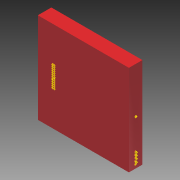
# Autodesk Inventor part: xM
Saved by Autodesk Inventor 2011 SP1 (Build 150282100, 282)
## iProperties
Created: 2011-06-13
Part Number: xM
Document SubType Name: Modeling
Designer: Andrew G. Meyer
Mass: 92.5046 g
Surface Area: 189.909 cm^2
Volume: 92.5046 cm^3
Density: 1 g/cm^3
Author: Andrew G. Meyer
Autodesk Inventor part; units mm, degrees
ref_plane "YZ Plane" through (0, 0, 0) normal (1, 0, 0) x (0, 1, 0)
ref_plane "XZ Plane" through (0, 0, 0) normal (0, 1, 0) x (-1, 0, 0)
ref_plane "XY Plane" through (0, 0, 0) normal (0, 0, 1) x (1, 0, 0)
sketch "Sketch1" plane through (0, 0, 0) normal (0, 0, 1) x (1, 0, 0)
  line L0 (-22.1557, 68.2637) -> (63.4423, 68.2637)
  line L1 (63.4423, 68.2637) -> (63.4423, -16.8263)
  line L2 (63.4423, -16.8263) -> (-22.1557, -16.8263)
  line L3 (-22.1557, -16.8263) -> (-22.1557, 68.2637)
  point P0 (0, 0)
  dimension "d0" = 85.09
  dimension "d1" = 85.598
  constraints: 8 end point, 2 parallel, 1 horizontal, 1 perpendicular
  measures "d0" distance of L2.end L0.start
  measures "d1" distance of L1.end L2.end
extrude "Extrusion1" add sketch "Sketch1" along normal blind 12.7
sketch "Sketch2" plane through (0, 0, 12.7) normal (0, 0, 1) x (1, 0, 0)
  line L0 (-22.1557, 68.2637) -> (63.4423, 68.2637) projected
  line L1 (-22.1557, -16.8263) -> (-22.1557, 68.2637) projected
  line L2 (63.4423, -16.8263) -> (-22.1557, -16.8263) projected
  line L3 (-9.4557, 36.5137) -> (-6.2807, 36.5137)
  line L4 (-6.2807, 36.5137) -> (-6.2807, 14.9237)
  line L5 (-6.2807, 14.9237) -> (-9.4557, 14.9237)
  line L6 (-9.4557, 14.9237) -> (-9.4557, 36.5137)
  point P0 (0, 0)
  dimension "d4" = 31.75
  dimension "d5" = 31.75
  dimension "d6" = 12.7
  dimension "d7" = 3.175
  constraints: 8 end point, 2 parallel, 1 horizontal, 1 perpendicular
  measures "d4" distance between parallel lines of L0 L3
  measures "d5" distance between parallel lines of L2 L5
  measures "d6" distance between parallel lines of L1 L6
  measures "d7" distance of L4.end L5.end
extrude "Extrusion2" cut sketch "Sketch2" against normal blind 0.254
sketch "Sketch3" plane through (0, 0, 12.446) normal (0, 0, 1) x (1, 0, 0)
  line L0 (-9.4557, 36.5137) -> (-9.4557, 14.9237) projected
  line L1 (-9.4557, 14.9237) -> (-6.2807, 14.9237) projected
  line L2 (-6.2807, 14.9237) -> (-7.7412, 14.9237)
  line L3 (-7.7412, 14.9237) -> (-7.7412, 16.3842)
  line L4 (-7.7412, 16.3842) -> (-6.2807, 16.3842)
  line L5 (-6.2807, 16.3842) -> (-6.2807, 14.9237)
  line L6 (-9.4557, 16.3842) -> (-7.9952, 16.3842)
  line L7 (-7.9952, 16.3842) -> (-7.9952, 14.9237)
  line L8 (-7.9952, 14.9237) -> (-9.4557, 14.9237)
  line L9 (-9.4557, 14.9237) -> (-9.4557, 16.3842)
  line L10 (-6.2807, 16.5112) -> (-7.7412, 16.5112)
  line L11 (-7.7412, 16.5112) -> (-7.7412, 17.9717)
  line L12 (-7.7412, 17.9717) -> (-6.2807, 17.9717)
  line L13 (-6.2807, 17.9717) -> (-6.2807, 16.5112)
  line L14 (-9.4557, 17.9717) -> (-7.9952, 17.9717)
  line L15 (-7.9952, 17.9717) -> (-7.9952, 16.5112)
  line L16 (-7.9952, 16.5112) -> (-9.4557, 16.5112)
  line L17 (-9.4557, 16.5112) -> (-9.4557, 17.9717)
  line L18 (-6.2807, 18.0987) -> (-7.7412, 18.0987)
  line L19 (-7.7412, 18.0987) -> (-7.7412, 19.5592)
  line L20 (-7.7412, 19.5592) -> (-6.2807, 19.5592)
  line L21 (-6.2807, 19.5592) -> (-6.2807, 18.0987)
  line L22 (-9.4557, 19.5592) -> (-7.9952, 19.5592)
  line L23 (-7.9952, 19.5592) -> (-7.9952, 18.0987)
  line L24 (-7.9952, 18.0987) -> (-9.4557, 18.0987)
  line L25 (-9.4557, 18.0987) -> (-9.4557, 19.5592)
  line L26 (-6.2807, 19.6862) -> (-7.7412, 19.6862)
  line L27 (-7.7412, 19.6862) -> (-7.7412, 21.1467)
  line L28 (-7.7412, 21.1467) -> (-6.2807, 21.1467)
  line L29 (-6.2807, 21.1467) -> (-6.2807, 19.6862)
  line L30 (-9.4557, 21.1467) -> (-7.9952, 21.1467)
  line L31 (-7.9952, 21.1467) -> (-7.9952, 19.6862)
  line L32 (-7.9952, 19.6862) -> (-9.4557, 19.6862)
  line L33 (-9.4557, 19.6862) -> (-9.4557, 21.1467)
  line L34 (-6.2807, 21.2737) -> (-7.7412, 21.2737)
  line L35 (-7.7412, 21.2737) -> (-7.7412, 22.7342)
  line L36 (-7.7412, 22.7342) -> (-6.2807, 22.7342)
  line L37 (-6.2807, 22.7342) -> (-6.2807, 21.2737)
  line L38 (-9.4557, 22.7342) -> (-7.9952, 22.7342)
  line L39 (-7.9952, 22.7342) -> (-7.9952, 21.2737)
  line L40 (-7.9952, 21.2737) -> (-9.4557, 21.2737)
  line L41 (-9.4557, 21.2737) -> (-9.4557, 22.7342)
  line L42 (-6.2807, 22.8612) -> (-7.7412, 22.8612)
  line L43 (-7.7412, 22.8612) -> (-7.7412, 24.3217)
  line L44 (-7.7412, 24.3217) -> (-6.2807, 24.3217)
  line L45 (-6.2807, 24.3217) -> (-6.2807, 22.8612)
  line L46 (-9.4557, 24.3217) -> (-7.9952, 24.3217)
  line L47 (-7.9952, 24.3217) -> (-7.9952, 22.8612)
  line L48 (-7.9952, 22.8612) -> (-9.4557, 22.8612)
  line L49 (-9.4557, 22.8612) -> (-9.4557, 24.3217)
  line L50 (-6.2807, 24.4487) -> (-7.7412, 24.4487)
  line L51 (-7.7412, 24.4487) -> (-7.7412, 25.9092)
  line L52 (-7.7412, 25.9092) -> (-6.2807, 25.9092)
  line L53 (-6.2807, 25.9092) -> (-6.2807, 24.4487)
  line L54 (-9.4557, 25.9092) -> (-7.9952, 25.9092)
  line L55 (-7.9952, 25.9092) -> (-7.9952, 24.4487)
  line L56 (-7.9952, 24.4487) -> (-9.4557, 24.4487)
  line L57 (-9.4557, 24.4487) -> (-9.4557, 25.9092)
  line L58 (-6.2807, 26.0362) -> (-7.7412, 26.0362)
  line L59 (-7.7412, 26.0362) -> (-7.7412, 27.4967)
  line L60 (-7.7412, 27.4967) -> (-6.2807, 27.4967)
  line L61 (-6.2807, 27.4967) -> (-6.2807, 26.0362)
  line L62 (-9.4557, 27.4967) -> (-7.9952, 27.4967)
  line L63 (-7.9952, 27.4967) -> (-7.9952, 26.0362)
  line L64 (-7.9952, 26.0362) -> (-9.4557, 26.0362)
  line L65 (-9.4557, 26.0362) -> (-9.4557, 27.4967)
  line L66 (-6.2807, 27.6237) -> (-7.7412, 27.6237)
  line L67 (-7.7412, 27.6237) -> (-7.7412, 29.0842)
  line L68 (-7.7412, 29.0842) -> (-6.2807, 29.0842)
  line L69 (-6.2807, 29.0842) -> (-6.2807, 27.6237)
  line L70 (-9.4557, 29.0842) -> (-7.9952, 29.0842)
  line L71 (-7.9952, 29.0842) -> (-7.9952, 27.6237)
  line L72 (-7.9952, 27.6237) -> (-9.4557, 27.6237)
  line L73 (-9.4557, 27.6237) -> (-9.4557, 29.0842)
  line L74 (-6.2807, 29.2112) -> (-7.7412, 29.2112)
  line L75 (-7.7412, 29.2112) -> (-7.7412, 30.6717)
  line L76 (-7.7412, 30.6717) -> (-6.2807, 30.6717)
  line L77 (-6.2807, 30.6717) -> (-6.2807, 29.2112)
  line L78 (-9.4557, 30.6717) -> (-7.9952, 30.6717)
  line L79 (-7.9952, 30.6717) -> (-7.9952, 29.2112)
  line L80 (-7.9952, 29.2112) -> (-9.4557, 29.2112)
  line L81 (-9.4557, 29.2112) -> (-9.4557, 30.6717)
  line L82 (-6.2807, 30.7987) -> (-7.7412, 30.7987)
  line L83 (-7.7412, 30.7987) -> (-7.7412, 32.2592)
  line L84 (-7.7412, 32.2592) -> (-6.2807, 32.2592)
  line L85 (-6.2807, 32.2592) -> (-6.2807, 30.7987)
  line L86 (-9.4557, 32.2592) -> (-7.9952, 32.2592)
  line L87 (-7.9952, 32.2592) -> (-7.9952, 30.7987)
  line L88 (-7.9952, 30.7987) -> (-9.4557, 30.7987)
  line L89 (-9.4557, 30.7987) -> (-9.4557, 32.2592)
  line L90 (-6.2807, 32.3862) -> (-7.7412, 32.3862)
  line L91 (-7.7412, 32.3862) -> (-7.7412, 33.8467)
  line L92 (-7.7412, 33.8467) -> (-6.2807, 33.8467)
  line L93 (-6.2807, 33.8467) -> (-6.2807, 32.3862)
  line L94 (-9.4557, 33.8467) -> (-7.9952, 33.8467)
  line L95 (-7.9952, 33.8467) -> (-7.9952, 32.3862)
  line L96 (-7.9952, 32.3862) -> (-9.4557, 32.3862)
  line L97 (-9.4557, 32.3862) -> (-9.4557, 33.8467)
  line L98 (-6.2807, 33.9737) -> (-7.7412, 33.9737)
  line L99 (-7.7412, 33.9737) -> (-7.7412, 35.4342)
  line L100 (-7.7412, 35.4342) -> (-6.2807, 35.4342)
  line L101 (-6.2807, 35.4342) -> (-6.2807, 33.9737)
  line L102 (-9.4557, 35.4342) -> (-7.9952, 35.4342)
  line L103 (-7.9952, 35.4342) -> (-7.9952, 33.9737)
  line L104 (-7.9952, 33.9737) -> (-9.4557, 33.9737)
  line L105 (-9.4557, 33.9737) -> (-9.4557, 35.4342)
  point P0 (0, 0)
  dimension "d10" = 0.254
  dimension "d13" = 1.5875
  constraints: 208 end point, 4 parallel, 3 equal length, 2 horizontal, 2 perpendicular, 2 point on line, 1 vertical, 192 other
  measures "d10" distance between parallel lines of L3 L7
  measures "d13" distance of L6.start L14.start
extrude "Extrusion3" add sketch "Sketch3" along normal blind 0.508
sketch "Sketch4" plane through (63.4423, -16.8263, 0) normal (1, 0, 0) x (0, 0, -1)
  line L0 (-12.7, 85.09) -> (-12.7, 0) projected
  line L1 (0, 0) -> (-12.7, 0) projected
  line L2 (0, 85.09) -> (0, 0) projected
  line L3 (0, 85.09) -> (-12.7, 85.09) projected
  circle A0 centre (-6.35, 42.545) radius 1.05
  circle A1 centre (-6.35, 42.545) radius 0.35
  line L4 (-6.35, 42.545) -> (-6.35, 0) construction
  line L5 (-6.35, 42.545) -> (-6.35, 85.09) construction
  line L6 (-6.35, 42.545) -> (0, 42.545) construction
  line L7 (-6.35, 42.545) -> (-12.7, 42.545) construction
  circle A2 centre (-6.35, 41.845) radius 0.25
  line L8 (-6.35, 41.845) -> (-6.35, 42.195) construction
  line L9 (-6.35, 41.845) -> (-6.35, 41.495) construction
  line L10 (-7.9375, 3.556) -> (-7.9375, 13.8995)
  line L11 (-6.579, 14.856) -> (-5.436, 14.4468)
  line L12 (-4.7625, 13.4902) -> (-4.7625, 3.9652)
  line L13 (-5.436, 3.0087) -> (-6.579, 2.5995)
  arc A3 (-7.9375, 3.556) -> (-6.579, 2.5995) centre (-6.9215, 3.556) ccw
  arc A4 (-5.436, 3.0087) -> (-4.7625, 3.9652) centre (-5.7785, 3.9652) ccw
  arc A5 (-6.579, 14.856) -> (-7.9375, 13.8995) centre (-6.9215, 13.8995) ccw
  arc A6 (-4.7625, 13.4902) -> (-5.436, 14.4468) centre (-5.7785, 13.4902) ccw
  circle A7 centre (-6.9215, 3.556) radius 0.6579
  circle A8 centre (-6.9215, 6.1419) radius 0.6579
  circle A9 centre (-6.9215, 8.7277) radius 0.6579
  circle A10 centre (-6.9215, 13.8995) radius 0.6579
  line L14 (-6.9215, 3.556) -> (-6.9215, 6.1419) construction
  line L15 (-6.9215, 6.1419) -> (-6.9215, 8.7277) construction
  circle A11 centre (-5.7785, 4.8489) radius 0.6579
  circle A12 centre (-6.9215, 11.3136) radius 0.6579
  circle A13 centre (-5.7785, 7.4348) radius 0.6579
  circle A14 centre (-5.7785, 10.0207) radius 0.6579
  circle A15 centre (-5.7785, 12.6066) radius 0.6579
  line L16 (-6.9215, 8.7277) -> (-6.9215, 11.3136) construction
  line L17 (-6.9215, 13.8995) -> (-6.9215, 11.3136) construction
  line L18 (-5.7785, 4.8489) -> (-5.7785, 7.4348) construction
  line L19 (-5.7785, 10.0207) -> (-5.7785, 7.4348) construction
  line L20 (-5.7785, 10.0207) -> (-5.7785, 12.6066) construction
  line L21 (-5.7785, 4.8489) -> (-6.9215, 4.8489) construction
  line L22 (-5.7785, 3.9652) -> (-5.7785, 4.8489) construction
  line L23 (-5.7785, 12.6066) -> (-5.7785, 13.0952) construction
  line L24 (-7.9375, 3.556) -> (-12.7, 3.556) construction
  line L25 (-4.7625, 3.9652) -> (0, 3.9652) construction
  point P0 (0, 16.8263)
  dimension "d20" = 2.1
  dimension "d21" = 0.7
  dimension "d22" = 0.5
  dimension "d23" = 109.7
  dimension "d24" = 1.016
  dimension "d25" = 109.7
  dimension "d26" = 3.175
  dimension "d27" = 9.525
  dimension "d28" = 1.27
  dimension "d29" = 2.54
  constraints: 44 end point, 14 centre point, 11 equal radius, 10 equal length, 8 point on circle, 8 tangent, 5 collinear, 5 midpoint, 5 point on line, 4 parallel, 4 perpendicular, 3 coincident, 2 vertical alignment, 4 other
  measures "d22" diameter of A2
  measures "d23" angle of L12 L13
  measures "d24" radius of A3
  measures "d25" angle of L12 L11
  measures "d26" distance between parallel lines of L12 L10
  measures "d27" distance of L12.start L12.end
  measures "d29" distance edge to line of A3 L1
extrude "Extrusion4" cut sketch "Sketch4" against normal blind 0.254 contours A0 | L10 A5 L11 A6 L12 A4 L13 A3
sketch "Sketch5" plane through (63.4423, -10.6845, 6.9215) normal (1, 0, 0) x (0, 0, -1)
  circle A0 centre (0, 0) radius 0.6579 construction
sketch "Sketch6" plane through (63.4423, -8.0986, 6.9215) normal (1, 0, 0) x (0, 0, -1)
  circle A0 centre (0, 0) radius 0.6579 construction
sketch "Sketch7" plane through (63.4423, -5.5127, 6.9215) normal (1, 0, 0) x (0, 0, -1)
  circle A0 centre (0, 0) radius 0.6579 construction
sketch "Sketch8" plane through (63.4423, -2.9269, 6.9215) normal (1, 0, 0) x (0, 0, -1)
  circle A0 centre (0, 0) radius 0.6579 construction
sketch "Sketch9" plane through (63.4423, -11.9774, 5.7785) normal (1, 0, 0) x (0, 0, -1)
  circle A0 centre (0, 0) radius 0.6579 construction
sketch "Sketch10" plane through (63.4423, -9.3915, 5.7785) normal (1, 0, 0) x (0, 0, -1)
  circle A0 centre (0, 0) radius 0.6579 construction
sketch "Sketch11" plane through (63.4423, -6.8057, 5.7785) normal (1, 0, 0) x (0, 0, -1)
  circle A0 centre (0, 0) radius 0.6579 construction
sketch "Sketch12" plane through (63.4423, -4.2198, 5.7785) normal (1, 0, 0) x (0, 0, -1)
  circle A0 centre (0, 0) radius 0.6579 construction
sketch "Sketch13" plane through (63.4423, 25.7187, 6.35) normal (1, 0, 0) x (0, 0, -1)
  circle A0 centre (0, 0) radius 0.35 construction
sketch "Sketch14" plane through (63.4423, 25.0187, 6.35) normal (1, 0, 0) x (0, 0, -1)
  circle A0 centre (0, 0) radius 0.25 construction
equation "\"d5\" = d4"
equation "\"d25\" = d23"
body "Solid1"
